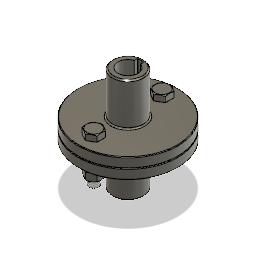
ParametricAssembly (Autodesk Fusion 360 design; units mm, degrees)
Autodesk Fusion 360 part; units mm, degrees
sketch "Sketch1" plane through (0, 0, 0) normal (0, 0, 1) x (1, 0, 0) in component "Полумуфта (16-11-1 УЗ ГОСТ 20761-96) v2"
  line L0 (0, 0) -> (0, 95.9076)
  line L1 (0, 42) -> (12.5, 42)
  line L2 (12.5, 42) -> (12.5, 9)
  line L3 (13.5, 8) -> (40, 8)
  line L4 (40, 8) -> (40, 0)
  line L5 (40, 0) -> (0, 0)
  line L6 (0, 2) -> (12.5, 2)
  line L7 (12.5, 2) -> (12.5, 0)
  arc A0 (12.5, 9) -> (13.5, 8) centre (13.5, 9) ccw
  dimension "d3" = 80
  dimension "d4" = 42
  dimension "d10" = 25
  dimension "d12" = 2
  dimension "d13" = 8
  dimension "d14" = 25
  dimension "d39" = 1
  constraint coincident L0.start L5.end
  constraint vertical L0
  constraint coincident L0 L1.start
  constraint perpendicular L0 L1
  constraint perpendicular L2 L3
  constraint perpendicular L3 L4
  constraint vertical L2
  constraint horizontal L5
  constraint coincident L0 L6.start
  constraint perpendicular L0 L6
  constraint coincident L5 L7.end
  constraint perpendicular L5 L7
  constraint tangent L2 A0
  constraint tangent L3 A0
  measures "d4" distance of L1 L5
  measures "d12" distance of L6.end L7.end
  measures "d13" distance of L3.end L4.end
  measures "d39" radius of A0
revolve "Revolve1" add sketch "Sketch1" angle 360 about axis through (0, 0, 0) along (0, 1, 0) contours L0 L1 L2 L3 L4 L5 L6 L7 A0 makes body 1 in component "Полумуфта (16-11-1 УЗ ГОСТ 20761-96) v2"
sketch "Sketch2" plane through (0, 42, 0) normal (0, 1, 0) x (-1, 0, 0) in component "Полумуфта (16-11-1 УЗ ГОСТ 20761-96) v2"
  circle A0 centre (0, 0) radius 12.5
  circle A1 centre (0, 0) radius 8
  line L0 (0, 0) -> (0, -40.0415) construction
  line L1 (2.5, -7.5993) -> (2.5, -10.1)
  line L2 (2.3, -10.3) -> (0, -10.3)
  line L3 (0, 0) -> (0, 8) construction
  line L4 (0, -10.3) -> (-2.3, -10.3)
  line L5 (-2.5, -10.1) -> (-2.5, -7.5993)
  arc A2 (2.3, -10.3) -> (2.5, -10.1) centre (2.3, -10.1) ccw
  arc A3 (-2.5, -10.1) -> (-2.3, -10.3) centre (-2.3, -10.1) ccw
  point P0 (2.5, -10.3)
  dimension "d17" = 16
  dimension "d21" = 2.5
  dimension "d24" = 18.3
  dimension "d42" = 0.2
  dimension "d43" = 0.2
  constraint coincident A0.centre A1.centre
  constraint vertical L0
  constraint coincident A1 L1.start
  constraint vertical L1
  constraint coincident L0 L2.end
  constraint horizontal L2
  constraint coincident A1 L3.end
  constraint parallel L0 L3
  constraint perpendicular L0 L4
  constraint coincident A1 L5.end
  constraint perpendicular L4 L5
  constraint coincident P0 L2
  constraint coincident P0 L1
  constraint tangent L2 A2
  constraint tangent L1 A2
  constraint tangent L4 A3
  constraint tangent L5 A3
  constraint equal L1 L5
  measures "d17" diameter of A1
  measures "d21" distance of P0 L2.end
  measures "d24" distance of L2.end L3.end
  measures "d42" radius of A2
  measures "d43" radius of A3
extrude "Extrude1" cut sketch "Sketch2" along normal mid plane 2000 contours A1 | A1 L1 L2 L4 L5 A2 A3 bodies 1 in component "Полумуфта (16-11-1 УЗ ГОСТ 20761-96) v2"
sketch "Sketch3" plane through (0, 8, 0) normal (0, 1, 0) x (-1, 0, 0) in component "Полумуфта (16-11-1 УЗ ГОСТ 20761-96) v2"
  circle A0 centre (0, 0) radius 40
  circle A1 centre (0, 0) radius 27.5 construction
  line L0 (0, -40) -> (0, 40) construction
  circle A2 centre (0, -27.5) radius 4
  circle A3 centre (0, 27.5) radius 4.5
  circle A4 centre (0, 0) radius 13.5
  dimension "d30" = 55
  dimension "d31" = 8
  dimension "d32" = 9
  constraint coincident A0.centre A1.centre
  constraint coincident A0 L0.start
  constraint coincident A0 L0.end
  constraint vertical L0
  constraint coincident A0.centre L0
  constraint coincident A1 A2.centre
  constraint coincident L0 A2.centre
  constraint coincident L0 A3.centre
  constraint coincident A1 A3.centre
  measures "d30" diameter of A1
  measures "d31" diameter of A2
  measures "d32" diameter of A3
extrude "Extrude2" cut sketch "Sketch3" along normal mid plane 2000 contours A2 | A3 bodies 1 in component "Полумуфта (16-11-1 УЗ ГОСТ 20761-96) v2"
chamfer "Chamfer1" distance 1 angle 45 1 edges at (-11.6541, 42, -4.5202) on bodies 1 in component "Полумуфта (16-11-1 УЗ ГОСТ 20761-96) v2"
chamfer "Chamfer2" distance 0.5 angle 45 4 edges at (4.1955, 8, 29.1273) (3.7293, 8, -26.0535) (-37.2931, 8, -14.4646) (-37.2931, 0, -14.4646) on bodies 1 in component "Полумуфта (16-11-1 УЗ ГОСТ 20761-96) v2"
sketch "Sketch1 (2)" plane through (0, 0, 0) normal (0, 0, 1) x (1, 0, 0) in component "Полумуфта (16-11-1 УЗ ГОСТ 20761-96) v2 (1)"
  line L0 (0, 0) -> (0, 95.9076)
  line L1 (0, 42) -> (12.5, 42)
  line L2 (12.5, 42) -> (12.5, 9)
  line L3 (13.5, 8) -> (40, 8)
  line L4 (40, 8) -> (40, 0)
  line L5 (40, 0) -> (0, 0)
  line L6 (0, 2) -> (12.5, 2)
  line L7 (12.5, 2) -> (12.5, 0)
  arc A0 (12.5, 9) -> (13.5, 8) centre (13.5, 9) ccw
  dimension "d3_1" = 80
  dimension "d4_1" = 42
  dimension "d10_1" = 25
  dimension "d12_1" = 2
  dimension "d13_1" = 8
  dimension "d14_1" = 25
  dimension "d39_1" = 1
  constraint coincident L0.start L5.end
  constraint vertical L0
  constraint coincident L0 L1.start
  constraint perpendicular L0 L1
  constraint perpendicular L2 L3
  constraint perpendicular L3 L4
  constraint vertical L2
  constraint horizontal L5
  constraint coincident L0 L6.start
  constraint perpendicular L0 L6
  constraint coincident L5 L7.end
  constraint perpendicular L5 L7
  constraint tangent L2 A0
  constraint tangent L3 A0
  measures "d4_1" distance of L1 L5
  measures "d12_1" distance of L6.end L7.end
  measures "d13_1" distance of L3.end L4.end
  measures "d39_1" radius of A0
revolve "Revolve1'" add sketch "Sketch1 (2)" angle 360 about axis through (0, 0, 0) along (0, 1, 0) separate body contours L0 L1 L2 L3 L4 L5 L6 L7 A0 makes body 2 in component "Полумуфта (16-11-1 УЗ ГОСТ 20761-96) v2 (1)"
sketch "Sketch2 (2)" plane through (0, 42, 0) normal (0, 1, 0) x (-1, 0, 0) in component "Полумуфта (16-11-1 УЗ ГОСТ 20761-96) v2 (1)"
  circle A0 centre (0, 0) radius 12.5
  circle A1 centre (0, 0) radius 8
  line L0 (0, 0) -> (0, -40.0415) construction
  line L1 (2.5, -7.5993) -> (2.5, -10.1)
  line L2 (2.3, -10.3) -> (0, -10.3)
  line L3 (0, 0) -> (0, 8) construction
  line L4 (0, -10.3) -> (-2.3, -10.3)
  line L5 (-2.5, -10.1) -> (-2.5, -7.5993)
  arc A2 (2.3, -10.3) -> (2.5, -10.1) centre (2.3, -10.1) ccw
  arc A3 (-2.5, -10.1) -> (-2.3, -10.3) centre (-2.3, -10.1) ccw
  point P0 (2.5, -10.3)
  dimension "d17_1" = 16
  dimension "d21_1" = 2.5
  dimension "d24_1" = 18.3
  dimension "d42_1" = 0.2
  dimension "d43_1" = 0.2
  constraint coincident A0.centre A1.centre
  constraint vertical L0
  constraint coincident A1 L1.start
  constraint vertical L1
  constraint coincident L0 L2.end
  constraint horizontal L2
  constraint coincident A1 L3.end
  constraint parallel L0 L3
  constraint perpendicular L0 L4
  constraint coincident A1 L5.end
  constraint perpendicular L4 L5
  constraint coincident P0 L2
  constraint coincident P0 L1
  constraint tangent L2 A2
  constraint tangent L1 A2
  constraint tangent L4 A3
  constraint tangent L5 A3
  constraint equal L1 L5
  measures "d17_1" diameter of A1
  measures "d21_1" distance of P0 L2.end
  measures "d24_1" distance of L2.end L3.end
  measures "d42_1" radius of A2
  measures "d43_1" radius of A3
extrude "Extrude1'" cut sketch "Sketch2 (2)" along normal mid plane 2000 contours A1 | A1 L1 L2 L4 L5 A2 A3 bodies 2 in component "Полумуфта (16-11-1 УЗ ГОСТ 20761-96) v2 (1)"
sketch "Sketch3 (2)" plane through (0, 8, 0) normal (0, 1, 0) x (-1, 0, 0) in component "Полумуфта (16-11-1 УЗ ГОСТ 20761-96) v2 (1)"
  circle A0 centre (0, 0) radius 40
  circle A1 centre (0, 0) radius 27.5 construction
  line L0 (0, -40) -> (0, 40) construction
  circle A2 centre (0, -27.5) radius 4
  circle A3 centre (0, 27.5) radius 4.5
  circle A4 centre (0, 0) radius 13.5
  dimension "d30_1" = 55
  dimension "d31_1" = 8
  dimension "d32_1" = 9
  constraint coincident A0.centre A1.centre
  constraint coincident A0 L0.start
  constraint coincident A0 L0.end
  constraint vertical L0
  constraint coincident A0.centre L0
  constraint coincident A1 A2.centre
  constraint coincident L0 A2.centre
  constraint coincident L0 A3.centre
  constraint coincident A1 A3.centre
  measures "d30_1" diameter of A1
  measures "d31_1" diameter of A2
  measures "d32_1" diameter of A3
extrude "Extrude2'" cut sketch "Sketch3 (2)" along normal mid plane 2000 contours A2 | A3 bodies 2 in component "Полумуфта (16-11-1 УЗ ГОСТ 20761-96) v2 (1)"
chamfer "Chamfer1'" distance 1 angle 45 1 edges at (-11.6541, 42, -4.5202) on bodies 2 in component "Полумуфта (16-11-1 УЗ ГОСТ 20761-96) v2 (1)"
chamfer "Chamfer2'" distance 0.5 angle 45 4 edges at (4.1955, 8, 29.1273) (3.7293, 8, -26.0535) (-37.2931, 8, -14.4646) (-37.2931, 0, -14.4646) on bodies 2 in component "Полумуфта (16-11-1 УЗ ГОСТ 20761-96) v2 (1)"
sketch "Sketch1 (3)" plane through (0, 0, 0) normal (0, 1, 0) x (1, 0, 0) in component "БОЛТ ГОСТ 7796 v10"
  line L0 (0, 6.9282) -> (-6, 3.4641)
  line L1 (-6, 3.4641) -> (-6, -3.4641)
  line L2 (-6, -3.4641) -> (0, -6.9282)
  line L3 (0, -6.9282) -> (6, -3.4641)
  line L4 (6, -3.4641) -> (6, 3.4641)
  line L5 (6, 3.4641) -> (0, 6.9282)
  dimension "d2" = 12
  constraint vertical L4
  measures "d2" distance of L1 L4
extrude "Extrude1''" add sketch "Sketch1 (3)" along normal blind 5 separate body makes body 3 in component "БОЛТ ГОСТ 7796 v10"
sketch "Sketch2 (3)" plane through (0, 0, 0) normal (1, 0, 0) x (0, 0, -1) in component "БОЛТ ГОСТ 7796 v10"
  line L0 (-5.718, 5) -> (-7.8414, 5)
  line L1 (-7.8414, 5) -> (-7.8414, 3.774)
  line L2 (-7.8414, 3.774) -> (-5.718, 5)
  line L3 (0, 0) -> (0, 6.8651) construction
  point P0 (-3.4641, 5)
  dimension "d10_2" = 5.718
  dimension "d11" = 30
  constraint horizontal L0
  constraint perpendicular L0 L1
  constraint coincident L3.start origin
  constraint vertical L3
  constraint coincident L0 P0
  measures "d10_2" distance of L0.start L3
  measures "d11" angle of L0 L2
revolve "Revolve1''" cut sketch "Sketch2 (3)" angle 360 about axis through (0, 0, 0) along (0, 1, 0) bodies 3 in component "БОЛТ ГОСТ 7796 v10"
sketch "Sketch3 (3)" plane through (0, 0, 0) normal (1, 0, 0) x (0, 0, -1) in component "БОЛТ ГОСТ 7796 v10"
  line L0 (0, 6.1991) -> (0, -30)
  line L1 (-4, 0) -> (-4, -30)
  line L2 (-4, -30) -> (0, -30)
  line L3 (-4, 0) -> (0, 0)
  dimension "d15_2" = 30
  dimension "d17_2" = 8
  constraint vertical L0
  constraint coincident L3.end L0
  constraint vertical L1
  constraint horizontal L2
  constraint coincident L3.end origin
  constraint horizontal L3
  measures "d15_2" distance of L1.start L1.end
revolve "Revolve2" add sketch "Sketch3 (3)" angle 360 about axis through (0, 6.1991, 0) along (0, -1, 0) bodies 3 in component "БОЛТ ГОСТ 7796 v10"
chamfer "Chamfer1''" distance 0.5 angle 45 1 edges at (-3.7293, -30, 1.4465) on bodies 3 in component "БОЛТ ГОСТ 7796 v10"
thread "Thread1" "ISO Metric profile 8.0 M8x1.25 6g" major diameter 7.866 minor diameter 6.4455 pitch 1.25 angle 60 resizes the face on face at (0.3983, -9.8333, 3.9801) from (0, -29.5, 0) to (0, -7.5, 0) on bodies 3 in component "БОЛТ ГОСТ 7796 v10"
sketch "Sketch1 (4)" plane through (0, 0, 0) normal (0, 1, 0) x (1, 0, 0) in component "Болт ГОСТ 7817 v9"
  line L0 (-6, 3.4641) -> (-6, -3.4641)
  line L1 (-6, -3.4641) -> (0, -6.9282)
  line L2 (0, -6.9282) -> (6, -3.4641)
  line L3 (6, -3.4641) -> (6, 3.4641)
  line L4 (6, 3.4641) -> (0, 6.9282)
  line L5 (0, 6.9282) -> (-6, 3.4641)
  dimension "d2_1" = 12
  constraint vertical L3
  measures "d2_1" distance of L0 L3
extrude "Extrude1'''" add sketch "Sketch1 (4)" along normal blind 5 separate body makes body 4 in component "Болт ГОСТ 7817 v9"
sketch "Sketch2 (4)" plane through (0, 0, 0) normal (1, 0, 0) x (0, 0, -1) in component "Болт ГОСТ 7817 v9"
  line L0 (5.718, 5) -> (8.8863, 5)
  line L1 (8.8863, 5) -> (8.8863, 3.1708)
  line L2 (8.8863, 3.1708) -> (5.718, 5)
  line L3 (0, 0) -> (0, 6.2268) construction
  point P0 (6.9282, 5)
  dimension "d6_1" = 5.718
  dimension "d7_1" = 30
  constraint horizontal L0
  constraint vertical L1
  constraint coincident L3.start origin
  constraint vertical L3
  constraint coincident L0 P0
  measures "d6_1" distance of L0.start L3
  measures "d7_1" angle of L0 L2
revolve "Revolve1'''" cut sketch "Sketch2 (4)" angle 360 about axis through (0, 0, 0) along (0, 1, 0) bodies 4 in component "Болт ГОСТ 7817 v9"
sketch "Sketch3 (4)" plane through (0, 0, 0) normal (1, 0, 0) x (0, 0, -1) in component "Болт ГОСТ 7817 v9"
  line L0 (0, 0) -> (0, -49.5853)
  line L1 (-4.5, -0.2) -> (-4.5, -20.8849)
  line L2 (-4.5, -20.8849) -> (-4, -21.7509)
  line L3 (-4, -21.7509) -> (-4, -34)
  line L4 (-4, -34) -> (-2.65, -34)
  line L5 (-2.65, -34) -> (-2.65, -35)
  line L6 (-2.65, -35) -> (0, -35)
  arc A0 (-4.5, -0.2) -> (-4.7, 0) centre (-4.7, -0.2) ccw
  line L7 (0, 0) -> (-4.7, 0)
  dimension "d17_3" = 35
  dimension "d19_2" = 9
  dimension "d20_3" = 8
  dimension "d21_3" = 1
  dimension "d22_1" = 30
  dimension "d25" = 5.3
  dimension "d26" = 0.2
  constraint coincident L0.start L7.start
  constraint vertical L0
  constraint parallel L0 L1
  constraint parallel L1 L3
  constraint perpendicular L3 L4
  constraint perpendicular L4 L5
  constraint coincident L0 L6.end
  constraint perpendicular L0 L6
  constraint tangent L1 A0
  constraint tangent A0 L7
  constraint horizontal L7
  measures "d17_3" distance of L0.start L6.end
  measures "d21_3" distance of L4.end L5.end
  measures "d22_1" angle of L1 L2
  measures "d26" radius of A0
revolve "Revolve2'" add sketch "Sketch3 (4)" angle 360 about axis through (0, 0, 0) along (0, -1, 0) bodies 4 in component "Болт ГОСТ 7817 v9"
sketch "Sketch4" plane through (0, 0, 0) normal (0, 0, 1) x (1, 0, 0) in component "Болт ГОСТ 7817 v9"
  line L0 (0, 0) -> (0, -35.5194) construction
  circle A0 centre (0, -29.5) radius 1
  dimension "d29" = 2
  dimension "d30_2" = 29.5
  constraint coincident L0.start origin
  constraint vertical L0
  constraint coincident L0 A0.centre
  measures "d29" diameter of A0
  measures "d30_2" distance of L0.start A0.centre
extrude "Extrude2''" cut sketch "Sketch4" along normal mid plane 200 bodies 4 in component "Болт ГОСТ 7817 v9"
thread "Thread1'" "ISO Metric profile 8.0 M8x1.25 6g" major diameter 7.866 minor diameter 6.4455 pitch 1.25 angle 60 resizes the face on face at (-1.496, -28.4009, 3.7097) on bodies 4 in component "Болт ГОСТ 7817 v9"
sketch "Sketch1 (5)" plane through (0, 0, 0) normal (0, 1, 0) x (1, 0, 0) in component "Гайка ГОСТ v9"
  line L0 (-6, 3.4641) -> (-6, -3.4641)
  line L1 (-6, -3.4641) -> (0, -6.9282)
  line L2 (0, -6.9282) -> (6, -3.4641)
  line L3 (6, -3.4641) -> (6, 3.4641)
  line L4 (6, 3.4641) -> (0, 6.9282)
  line L5 (0, 6.9282) -> (-6, 3.4641)
  circle A0 centre (0, 0) radius 4
  dimension "d1" = 12
  dimension "d4_3" = 8
  constraint coincident A0.centre origin
  constraint vertical L3
  constraint vertical L0
  measures "d1" distance of L0 L3
  measures "d4_3" diameter of A0
extrude "Extrude1''''" add sketch "Sketch1 (5)" along normal blind 6.5 separate body makes body 5 in component "Гайка ГОСТ v9"
sketch "Sketch3 (5)" plane through (0, 0, 0) normal (1, 0, 0) x (0, 0, -1) in component "Гайка ГОСТ v9"
  line L0 (-5.718, 6.5) -> (-7.7165, 6.5)
  line L1 (-7.7165, 6.5) -> (-7.7165, 5.3462)
  line L2 (-7.7165, 5.3462) -> (-5.718, 6.5)
  line L3 (0, 0) -> (0, 8.4615)
  point P0 (0, 6.5)
  point P1 (-6.9282, 6.5)
  dimension "d9" = 5.718
  dimension "d10_3" = 30
  dimension "d11_1" = 1.1538
  constraint horizontal L0
  constraint perpendicular L0 L1
  constraint coincident L3.start origin
  constraint perpendicular L0 L3
  constraint coincident L0 P1
  measures "d9" distance of L0.start L3
  measures "d10_3" angle of L0 L2
  measures "d11_1" distance of L0.end L1.end
revolve "Revolve1''''" cut sketch "Sketch3 (5)" angle 360 about axis through (0, 0, 0) along (0, 1, 0) bodies 5 in component "Гайка ГОСТ v9"
ref_plane "WorkPlane1" through (0, 3.25, 0) normal (0, -1, 0) x (-1, 0, 0) in component "Гайка ГОСТ v9"
mirror "Mirror1" about plane through (0, 3.25, 0) normal (0, -1, 0) of 1 faces at (-5.3401, 6.1286, 3.4569) on bodies 5 in component "Гайка ГОСТ v9"
thread "Thread1''" "ISO Metric profile 8.0 M8x1.25 6H" major diameter 8.17 minor diameter 6.7795 pitch 1.25 angle 60 resizes the face on face at (3.9801, 4.3333, 0.3983) on bodies 5 in component "Гайка ГОСТ v9"
chamfer "Chamfer1'''" distance 0.5 angle 45 2 edges at (-3.1604, 6.5, -1.2258) (-3.1604, 0, -1.2258) 1 faces at (3.3729, 4.3333, 0.3375) on bodies 5 in component "Гайка ГОСТ v9"
sketch "Sketch1 (6)" plane through (0, 0, 0) normal (0, 1, 0) x (1, 0, 0) in component "Гайка ГОСТ v9 (1)"
  line L0 (-6, 3.4641) -> (-6, -3.4641)
  line L1 (-6, -3.4641) -> (0, -6.9282)
  line L2 (0, -6.9282) -> (6, -3.4641)
  line L3 (6, -3.4641) -> (6, 3.4641)
  line L4 (6, 3.4641) -> (0, 6.9282)
  line L5 (0, 6.9282) -> (-6, 3.4641)
  circle A0 centre (0, 0) radius 4
  dimension "d1_1" = 12
  dimension "d4_4" = 8
  constraint coincident A0.centre origin
  constraint vertical L3
  constraint vertical L0
  measures "d1_1" distance of L0 L3
  measures "d4_4" diameter of A0
extrude "Extrude1'''''" add sketch "Sketch1 (6)" along normal blind 6.5 separate body makes body 6 in component "Гайка ГОСТ v9 (1)"
sketch "Sketch3 (6)" plane through (0, 0, 0) normal (1, 0, 0) x (0, 0, -1) in component "Гайка ГОСТ v9 (1)"
  line L0 (-5.718, 6.5) -> (-7.7165, 6.5)
  line L1 (-7.7165, 6.5) -> (-7.7165, 5.3462)
  line L2 (-7.7165, 5.3462) -> (-5.718, 6.5)
  line L3 (0, 0) -> (0, 8.4615)
  point P0 (0, 6.5)
  point P1 (-6.9282, 6.5)
  dimension "d9_1" = 5.718
  dimension "d10_4" = 30
  dimension "d11_2" = 1.1538
  constraint horizontal L0
  constraint perpendicular L0 L1
  constraint coincident L3.start origin
  constraint perpendicular L0 L3
  constraint coincident L0 P1
  measures "d9_1" distance of L0.start L3
  measures "d10_4" angle of L0 L2
  measures "d11_2" distance of L0.end L1.end
revolve "Revolve1'''''" cut sketch "Sketch3 (6)" angle 360 about axis through (0, 0, 0) along (0, 1, 0) bodies 6 in component "Гайка ГОСТ v9 (1)"
ref_plane "WorkPlane1" through (0, 3.25, 0) normal (0, -1, 0) x (-1, 0, 0) in component "Гайка ГОСТ v9 (1)"
mirror "Mirror1'" about plane through (0, 3.25, 0) normal (0, -1, 0) of 1 faces at (-5.3401, 6.1286, 3.4569) on bodies 6 in component "Гайка ГОСТ v9 (1)"
thread "Thread1'''" "ISO Metric profile 8.0 M8x1.25 6H" major diameter 8.17 minor diameter 6.7795 pitch 1.25 angle 60 resizes the face on face at (3.9801, 4.3333, 0.3983) on bodies 6 in component "Гайка ГОСТ v9 (1)"
chamfer "Chamfer1''''" distance 0.5 angle 45 2 edges at (-3.1604, 6.5, -1.2258) (-3.1604, 0, -1.2258) 1 faces at (3.3729, 4.3333, 0.3375) on bodies 6 in component "Гайка ГОСТ v9 (1)"
component "Полумуфта (16-11-1 УЗ ГОСТ 20761-96) v2" placed x (1, 0, 0) y (0, 1, 0) z (0, 0, 1) at (0, 0, 0)
component "БОЛТ ГОСТ 7796 v10" placed x (1, 0, 0) y (0, 1, 0) z (0, 0, 1) at (0, 8.567, -27.5)
component "Болт ГОСТ 7817 v9" placed x (1, 0, 0) y (0, 1, 0) z (0, 0, 1) at (0, 8.5, 27.5)
component "Гайка ГОСТ v9" placed x (1, 0, 0) y (0, 1, 0) z (0, 0, 1) at (0, -15, -27.5)
component "Гайка ГОСТ v9 (1)" placed x (1, 0, 0) y (0, 1, 0) z (0, 0, 1) at (0, -19.7, 27.5)
component "Полумуфта (16-11-1 УЗ ГОСТ 20761-96) v2 (1)" placed x (-1, 0, 0) y (0, -1, 0) z (0, 0, 1) at (0, 0, 0)
equation "DHC = 80 mm"
equation "LHC = 42 mm"
equation "d3 = DHC"
equation "d4 = LHC"
equation "l_1HC = 8 mm"
equation "l_2HC = 2 mm"
equation "d_2HC = 25 mm"
equation "d_1HC = 16 mm"
equation "d10 = dHC"
equation "d12 = l_2HC"
equation "d13 = l_1HC"
equation "d14 = d_2HC"
equation "dHC = 25 mm"
equation "d17 = d_1HC"
equation "ext_all_HC = 1000 mm"
equation "d19 = ext_all_HC"
equation "d21 = B_HC"
equation "B_HC = 2.5 mm"
equation "H_HC = 18.3 mm"
equation "d24 = H_HC"
equation "d_3HC = 8 mm"
equation "d_4HC = 9 mm"
equation "D_2HC = 55 mm"
equation "b_1HC = 1 mm"
equation "b_2HC = 0.5 mm"
equation "d30 = D_2HC"
equation "d31 = d_3HC"
equation "d32 = d_4HC"
equation "d33 = ext_all_HC"
equation "d37 = b_1HC"
equation "R_1HC = 1 mm"
equation "d39 = R_1HC"
equation "d40 = b_2HC"
equation "R_HC = 0.2 mm"
equation "d42 = R_HC"
equation "d43 = R_HC"
equation "DHC_1 = 80 mm"
equation "LHC_1 = 42 mm"
equation "d3_1 = DHC_1"
equation "d4_1 = LHC_1"
equation "l_1HC_1 = 8 mm"
equation "l_2HC_1 = 2 mm"
equation "d_2HC_1 = 25 mm"
equation "d_1HC_1 = 16 mm"
equation "d10_1 = dHC_1"
equation "d12_1 = l_2HC_1"
equation "d13_1 = l_1HC_1"
equation "d14_1 = d_2HC_1"
equation "dHC_1 = 25 mm"
equation "d17_1 = d_1HC_1"
equation "ext_all_HC_1 = 1000 mm"
equation "d19_1 = ext_all_HC_1"
equation "d21_1 = B_HC_1"
equation "B_HC_1 = 2.5 mm"
equation "H_HC_1 = 18.3 mm"
equation "d24_1 = H_HC_1"
equation "d_3HC_1 = 8 mm"
equation "d_4HC_1 = 9 mm"
equation "D_2HC_1 = 55 mm"
equation "b_1HC_1 = 1 mm"
equation "b_2HC_1 = 0.5 mm"
equation "d30_1 = D_2HC_1"
equation "d31_1 = d_3HC_1"
equation "d32_1 = d_4HC_1"
equation "d33_1 = ext_all_HC_1"
equation "d37_1 = b_1HC_1"
equation "R_1HC_1 = 1 mm"
equation "d39_1 = R_1HC_1"
equation "d40_1 = b_2HC_1"
equation "R_HC_1 = 0.2 mm"
equation "d42_1 = R_HC_1"
equation "d43_1 = R_HC_1"
equation "S_bolt2 = 12 mm"
equation "d2 = S_bolt2"
equation "d_bolt2 = 8 mm"
equation "m_bolt2 = 5 mm"
equation "d6 = m_bolt2"
equation "D_bolt2 = 5.718 mm"
equation "d10_2 = D_bolt2"
equation "l1_bolt2 = 30 mm"
equation "b_bolt2 = 22 mm"
equation "d15_2 = l1_bolt2"
equation "d17_2 = d_bolt2"
equation "chm_bolt2 = 0.5 mm"
equation "d20_2 = chm_bolt2"
equation "thr_bolt2 = 8 mm"
equation "S_bolt = 12 mm"
equation "d2_1 = S_bolt"
equation "m_bolt = 5 mm"
equation "d4_2 = m_bolt"
equation "d6_1 = ( S_bolt * 0.953 ) / 2"
equation "L_bolt = 35 mm"
equation "l1_bolt = 29.5 mm"
equation "l2_bolt = 20.5 mm"
equation "d_bolt = 8 mm"
equation "d1_bolt = 9 mm"
equation "R_bolt = 0.2 mm"
equation "l3_bolt = 1 mm"
equation "d17_3 = L_bolt"
equation "d19_2 = d1_bolt"
equation "d20_3 = d_bolt"
equation "d21_3 = l3_bolt"
equation "d3_bolt = 5.3 mm"
equation "d4_bolt = 2 mm"
equation "d25 = d3_bolt"
equation "d26 = R_bolt"
equation "ext_all_bolt = 100 mm"
equation "d29 = d4_bolt"
equation "d30_2 = l1_bolt"
equation "d31_2 = ext_all_bolt"
equation "d1 = S_nut"
equation "S_nut = 12 mm"
equation "d_nut = 8 mm"
equation "d4_3 = d_nut"
equation "k_nut = 6.5 mm"
equation "d6_2 = k_nut"
equation "d9 = ( 0.953 * S_nut ) / 2"
equation "d13_2 = -k_nut / 2"
equation "ch_nut = 0.5 mm"
equation "d17_4 = ch_nut"
equation "d1_1 = S_nut_1"
equation "S_nut_1 = 12.0 mm"
equation "d_nut_1 = 8.0 mm"
equation "d4_4 = d_nut_1"
equation "k_nut_1 = 6.5 mm"
equation "d6_3 = k_nut_1"
equation "d9_1 = ( 0.953 * S_nut_1 ) / 2"
equation "d13_3 = -k_nut_1 / 2"
equation "ch_nut_1 = 0.5 mm"
equation "d17_5 = ch_nut_1"
equation "offset = -21 mm"
equation "angle = 180 deg"
